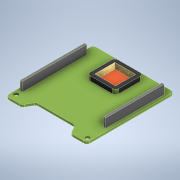
# Autodesk Inventor part: mti_3
Saved by Autodesk Inventor 2022 (Build 260153000, 153)
## iProperties
Created: 2021-10-11
Part Number: mti_3
Material: Generic
Document SubType Name: Modeling
Designer: skcre
Density: 1 g/cm^3
Appearance: Olive Green
Author: skcre
Autodesk Inventor part; units mm, degrees
ref_plane "YZ Plane" through (0, 0, 0) normal (1, 0, 0) x (0, 1, 0)
ref_plane "XZ Plane" through (0, 0, 0) normal (0, 1, 0) x (-1, 0, 0)
ref_plane "XY Plane" through (0, 0, 0) normal (0, 0, 1) x (1, 0, 0)
sketch "Sketch1" plane through (0, 0, 0) normal (0, 1, 0) x (-1, 0, 0)
  line L0 (-26.67, -28.76) -> (26.67, -28.76)
  line L1 (26.67, -28.76) -> (26.67, 28.76)
  line L2 (26.67, 28.76) -> (-26.67, 28.76)
  line L3 (-26.67, 28.76) -> (-26.67, -28.76)
  line L4 (-26.67, -28.76) -> (26.67, 28.76) construction
  line L5 (26.67, -28.76) -> (-26.67, 28.76) construction
  circle A0 centre (-24.13, 25.85) radius 1.5
  circle A1 centre (24.13, 24.58) radius 1.5
  circle A2 centre (-19.05, -26.25) radius 1.5
  point P0 (0, 0)
  point P1 (0, 0)
  dimension "d0" = 53.34
  dimension "d1" = 57.52
  dimension "d2" = 3
  dimension "d3" = 3
  dimension "d4" = 3
  dimension "d5" = 2.54
  dimension "d6" = 2.91
  dimension "d7" = 50.8
  dimension "d8" = 4.18
  dimension "d9" = 2.51
  dimension "d10" = 7.62
  constraints: 12 end point, 3 centre point, 2 midpoint, 2 parallel, 1 coincident, 1 horizontal, 1 perpendicular
  measures "d0" distance of L0.start L0.end
  measures "d1" distance of L2.end L0.start
  measures "d2" diameter of A0
  measures "d3" diameter of A1
  measures "d4" diameter of A2
  measures "d5" distance from line of L3 A0.centre
  measures "d6" distance from line of L2 A0.centre
  measures "d7" distance from line of L3 A1.centre
  measures "d8" distance from line of L2 A1.centre
  measures "d9" distance from line of L0 A2.centre
  measures "d10" distance from line of L3 A2.centre
extrude "Extrusion1" add sketch "Sketch1" along normal blind 1.5
sketch "Sketch2" plane through (0, 1.5, 0) normal (0, 1, 0) x (1, 0, 0)
  line L0 (-26.67, 28.76) -> (-26.67, -28.76) projected
  line L1 (-26.67, -28.76) -> (26.67, -28.76) projected
  line L2 (26.67, -28.76) -> (26.67, 28.76) projected
  line L3 (26.67, 28.76) -> (-26.67, 28.76) projected
  circle A0 centre (24.13, -25.85) radius 1.5 projected
  circle A1 centre (-24.13, -24.58) radius 1.5 projected
  circle A2 centre (19.05, 26.25) radius 1.5 projected
  line L4 (-26.67, -28.76) -> (26.67, -28.76) projected
  line L5 (0, -28.76) -> (0, 28.76)
  line L6 (9.3688, 25.76) -> (-9.3688, 25.76)
  line L7 (-9.3688, 25.76) -> (-9.3688, 7.4756)
  line L8 (-9.3688, 7.4756) -> (9.3688, 7.4756)
  line L9 (9.3688, 7.4756) -> (9.3688, 25.76)
  line L10 (9.3688, 25.76) -> (-9.3688, 7.4756) construction
  line L11 (-9.3688, 25.76) -> (9.3688, 7.4756) construction
  point P0 (0, 0)
  point P1 (0, 16.6178)
  dimension "d13" = 36.0388
  dimension "d14" = 3
  constraints: 14 end point, 4 midpoint, 2 parallel, 1 horizontal, 1 perpendicular, 1 point on line
  measures "d13" distance between parallel lines of L2 L7
  measures "d14" distance between parallel lines of L3 L6
extrude "Extrusion2" add sketch "Sketch2" along normal blind 3 contours L6 L9 L8 L5 | L5 L8 L7 L6
sketch "Sketch3" plane through (0, 1.5, 0) normal (0, 1, 0) x (1, 0, 0)
  line L0 (9.3688, 25.76) -> (9.3688, 7.4756) projected
  line L1 (9.3688, 7.4756) -> (-9.3688, 7.4756) projected
  line L2 (-9.3688, 7.4756) -> (-9.3688, 25.76) projected
  line L3 (-9.3688, 25.76) -> (9.3688, 25.76) projected
  line L4 (-26.67, 28.76) -> (-26.67, -28.76) projected
  line L5 (-26.67, -28.76) -> (26.67, -28.76) projected
  line L6 (26.67, -28.76) -> (26.67, 28.76) projected
  line L7 (26.67, 28.76) -> (-26.67, 28.76) projected
  circle A0 centre (24.13, -25.85) radius 1.5 projected
  circle A1 centre (-24.13, -24.58) radius 1.5 projected
  circle A2 centre (19.05, 26.25) radius 1.5 projected
  circle A3 centre (24.13, -25.85) radius 1.5 projected
  line L8 (24.13, -25.85) -> (24.13, 28.76)
  line L9 (26.67, 28.76) -> (-26.67, 28.76) projected
  line L10 (-24.13, -24.58) -> (-24.13, 28.76)
  line L11 (24.88, 24.099) -> (23.38, 24.099)
  line L12 (23.38, 24.099) -> (23.38, -14.4594)
  line L13 (23.38, -14.4594) -> (24.88, -14.4594)
  line L14 (24.88, -14.4594) -> (24.88, 24.099)
  line L15 (24.88, 24.099) -> (23.38, -14.4594) construction
  line L16 (23.38, 24.099) -> (24.88, -14.4594) construction
  line L17 (-24.88, 21.2829) -> (-23.38, 21.2829)
  line L18 (-23.38, 21.2829) -> (-23.38, -21.2829)
  line L19 (-23.38, -21.2829) -> (-24.88, -21.2829)
  line L20 (-24.88, -21.2829) -> (-24.88, 21.2829)
  line L21 (-24.88, 21.2829) -> (-23.38, -21.2829) construction
  line L22 (-23.38, 21.2829) -> (-24.88, -21.2829) construction
  point P0 (0, 0)
  point P1 (24.13, 4.8198)
  point P2 (-24.13, 0)
  dimension "d17" = 1.5
  dimension "d18" = 1.5
  constraints: 28 end point, 4 midpoint, 4 parallel, 4 perpendicular, 4 point on line, 2 horizontal
  measures "d17" distance of L12.end L13.end
  measures "d18" distance of L18.end L19.end
extrude "Extrusion3" add sketch "Sketch3" along normal blind 6 contours L11 L14 L13 L8 | L8 L13 L12 L11 | L17 L18 L19 L10 | L10 L19 L20 L17
sketch "Sketch4" plane through (0, 4.5, 0) normal (0, 1, 0) x (1, 0, 0)
  line L0 (9.3688, 25.76) -> (-9.3688, 25.76) projected
  line L1 (-9.3688, 25.76) -> (-9.3688, 7.4756) projected
  line L2 (-9.3688, 7.4756) -> (9.3688, 7.4756) projected
  line L3 (9.3688, 7.4756) -> (9.3688, 25.76) projected
  line L4 (4.8688, 11.9756) -> (-4.8688, 11.9756)
  line L5 (-4.8688, 11.9756) -> (-4.8688, 21.26)
  line L6 (-4.8688, 21.26) -> (4.8688, 21.26)
  line L7 (4.8688, 21.26) -> (4.8688, 11.9756)
  point P0 (0, 0)
  dimension "d21" = 4.5
  constraints: 8 end point, 3 other
  measures "d21" distance between parallel lines of L2 L4
extrude "Extrusion4" cut sketch "Sketch4" against normal blind 2 contours L4 L5 L6 L7
chamfer "Chamfer1" distance 2 angle 45 4 edges at (0, 4.5, -11.9756) (-4.8688, 4.5, -16.6178) (0, 4.5, -21.26) (4.8688, 4.5, -16.6178)
sketch "Sketch5" plane through (0, 1.5, 0) normal (0, 1, 0) x (1, 0, 0)
  line L0 (-26.67, -28.76) -> (26.67, -28.76) projected
  line L1 (-16.2954, -28.76) -> (-12.7903, -22.5498)
  line L2 (-12.7903, -22.5498) -> (0, -22.5498)
  line L3 (12.7903, -22.5498) -> (16.2954, -28.76)
  line L4 (0, -28.76) -> (0, -13.7349)
  line L5 (0, -22.5498) -> (12.7903, -22.5498)
  point P0 (0, 0)
  constraints: 10 end point, 3 point on line, 2 equal length, 2 parallel, 1 midpoint, 1 vertical
extrude "Extrusion5" cut sketch "Sketch5" against normal through all
fillet "Fillet1" radius 2 8 edges at (26.67, 0.75, -28.76) (-26.67, 0.75, -28.76) (-26.67, 0.75, 28.76) (-16.2954, 0.75, 28.76) (-12.7903, 0.75, 22.5498) (12.7903, 0.75, 22.5498) (16.2954, 0.75, 28.76) (26.67, 0.75, 28.76)
fillet "Fillet2" radius 2 4 edges at (9.3688, 3, -25.76) (9.3688, 3, -7.4756) (-9.3688, 3, -7.4756) (-9.3688, 3, -25.76)
body "Solid1"
